slot_gauge (Autodesk Fusion 360 design; units mm, degrees)
part number: 2026-09-02-15-56-11-666
Autodesk Fusion 360 part; units mm, degrees
sketch "Gauge plate" plane through (0, 0, 0) normal (0, 1, 0) x (1, 0, 0)
  line L0 (0, 0) -> (5, 0)
  line L1 (5, 0) -> (5, -90)
  line L2 (5, -90) -> (0, -90)
  line L3 (0, -90) -> (0, 0)
extrude "Gauge plate (1)" add sketch "Gauge plate" along normal mid plane 24
sketch "Hook profile" plane through (0, 0, 0) normal (0, 1, 0) x (1, 0, 0)
  line L0 (0, -88) -> (-8.3, -88)
  line L1 (-8.3, -88) -> (-8.3, -71)
  line L2 (-8.3, -71) -> (-5.3, -71)
  line L3 (-5.3, -71) -> (-3.8, -72.5)
  line L4 (-3.8, -72.5) -> (-3.8, -83)
  line L5 (-3.8, -83) -> (0, -83)
  line L6 (0, -83) -> (0, -88)
  dimension "d38" = 88
  dimension "d39" = 8.3
  dimension "d40" = 3.8
  dimension "d41" = 5
  dimension "d42" = 10.5
  dimension "d43" = 1.5
  dimension "d44" = 1.5
  constraint horizontal L0
  constraint horizontal L2
  constraint horizontal L5
  constraint vertical L1
  constraint vertical L4
  constraint vertical L6
  constraint coincident origin L6
  measures "d38" vertical distance of origin L0.start
  measures "d39" horizontal distance of L0.start L0.end
  measures "d40" horizontal distance of L4.end L5.end
  measures "d41" vertical distance of L0.start L5.end
  measures "d42" vertical distance of L3.end L4.end
  measures "d43" horizontal distance of L2.end L3.end
  measures "d44" vertical distance of L2.end L3.end
extrude "Hook profile (1)" add sketch "Hook profile" along normal mid plane 2.4
pattern_linear "Hook rows" count 4 spacing 25.4 along (0, 0, -1) count 3 spacing 0 along (0, 0, 1) of "Hook profile (1)"
equation "bracketWidth = 24.0 mm" comment "drives the model; safe to edit live in Fusion"
equation "couponWidth = 8.0 mm" comment "drives the model; safe to edit live in Fusion"
equation "hookTabWidth = 2.4 mm" comment "drives the model; safe to edit live in Fusion"
equation "slotHeight = 19.05 mm" comment "reference only â edit scripts/build_rod_bracket.py and rebuild"
equation "slotPitchVertical = 25.4 mm" comment "drives the model; safe to edit live in Fusion"
equation "slotWidth = 3.2 mm" comment "reference only â edit scripts/build_rod_bracket.py and rebuild"
equation "faceMetalThickness = 2.0 mm" comment "drives the model; safe to edit live in Fusion"
equation "hookThroat = faceMetalThickness + 1.8 mm" comment "drives the model; safe to edit live in Fusion"
equation "hookNeckHeight = 5.0 mm" comment "drives the model; safe to edit live in Fusion"
equation "hookLipThickness = 4.5 mm" comment "drives the model; safe to edit live in Fusion"
equation "hookLipDrop = 12.0 mm" comment "drives the model; safe to edit live in Fusion"
equation "plateThickness = 6.0 mm" comment "reference only â edit scripts/build_rod_bracket.py and rebuild"
equation "plateHeight = 90.0 mm" comment "reference only â edit scripts/build_rod_bracket.py and rebuild"
equation "gaugePlateThickness = 5.0 mm" comment "reference only â edit scripts/build_rod_bracket.py and rebuild"
equation "rodOuterDiameter = 33.4 mm" comment "reference only â edit scripts/build_rod_bracket.py and rebuild"
equation "saddleClearance = 0.8 mm" comment "reference only â edit scripts/build_rod_bracket.py and rebuild"
equation "saddleWall = 6.0 mm" comment "reference only â edit scripts/build_rod_bracket.py and rebuild"
equation "rearRodStandoff = 70.0 mm" comment "reference only â edit scripts/build_rod_bracket.py and rebuild"
equation "rodSpacing = 80.0 mm" comment "reference only â edit scripts/build_rod_bracket.py and rebuild"
equation "memberWidth = 14.0 mm" comment "reference only â edit scripts/build_rod_bracket.py and rebuild"
equation "hookLipChamfer = 1.5 mm" comment "drives the model; safe to edit live in Fusion"
equation "topHookNeckTop = 88.0 mm" comment "drives the model; safe to edit live in Fusion"
equation "hookRows = 4" comment "drives the model; safe to edit live in Fusion"
equation "d36 = bracketWidth"
equation "d38 = topHookNeckTop"
equation "d39 = hookThroat + hookLipThickness"
equation "d40 = hookThroat"
equation "d41 = hookNeckHeight"
equation "d42 = hookLipDrop - hookLipChamfer"
equation "d43 = hookLipChamfer"
equation "d44 = hookLipChamfer"
equation "d45 = hookTabWidth"
equation "d47 = hookRows"
equation "d49 = -slotPitchVertical"
named bodies: "slot_gauge"
